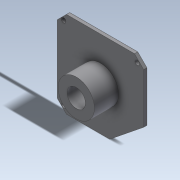
# Autodesk Inventor part: Arducam
Saved by Autodesk Inventor 2020 (Build 240168000, 168)
## iProperties
Created: 2020-11-17
Part Number: Arducam
Material: Generic
Document SubType Name: Modeling
Designer: valer
Density: 1 g/cm^3
Appearance: Default
Author: valer
Autodesk Inventor part; units mm, degrees
ref_plane "YZ Plane" through (0, 0, 0) normal (1, 0, 0) x (0, 1, 0)
ref_plane "XZ Plane" through (0, 0, 0) normal (0, 1, 0) x (-1, 0, 0)
ref_plane "XY Plane" through (0, 0, 0) normal (0, 0, 1) x (1, 0, 0)
sketch "Base" plane through (0, 0, 0) normal (0, 0, 1) x (1, 0, 0)
  line L0 (-20, 20) -> (20, 20)
  line L1 (20, 20) -> (20, -20)
  line L2 (20, -20) -> (-20, -20)
  line L3 (-20, -20) -> (-20, 20)
  line L4 (-15.74, 20) -> (-20, 15.74)
  line L5 (15.74, 20) -> (20, 15.74)
  line L6 (-17.02, 17.02) -> (17.02, 17.02) construction
  line L7 (17.02, 17.02) -> (17.02, -17.02) construction
  line L8 (17.02, -17.02) -> (-17.02, -17.02) construction
  line L9 (-17.02, -17.02) -> (-17.02, 17.02) construction
  line L10 (-17.02, 17.02) -> (17.02, -17.02) construction
  line L11 (17.02, 17.02) -> (-17.02, -17.02) construction
  circle A0 centre (0, 0) radius 8.4
  circle A1 centre (17.02, 17.02) radius 1.05
  circle A2 centre (-17.02, 17.02) radius 1.05
  circle A3 centre (-17.02, -17.02) radius 1.05
  circle A4 centre (17.02, -17.02) radius 1.05
  line L12 (-20, -15.74) -> (-15.74, -20)
  line L13 (20, -15.74) -> (15.74, -20)
  point P0 (0, 0)
  point P1 (0, 0)
  dimension "d0" = 40
  dimension "d1" = 40
  dimension "d2" = 135
  dimension "d3" = 135
  dimension "d4" = 31.48
  dimension "d5" = 34.04
  dimension "d6" = 2.98
  dimension "d7" = 2.98
  dimension "d8" = 2.98
  dimension "d9" = 2.98
  dimension "d10" = 16.8
  dimension "d11" = 2.1
  dimension "d12" = 135
  dimension "d13" = 135
  dimension "d14" = 31.48
  dimension "d15" = 34.04
  dimension "d16" = 31.48
  constraints: 28 end point, 8 point on line, 5 centre point, 5 coincident, 5 perpendicular, 4 parallel, 3 equal radius, 2 horizontal, 2 midpoint
  measures "d0" distance of L0.start L0.end
  measures "d1" distance of L2.end L0.start
  measures "d2" angle of L0 L4
  measures "d3" angle of L0 L5
  measures "d4" distance of L5.start L4.start
  measures "d5" distance of L6.start L6.end
  measures "d6" distance between parallel lines of L3 L9
  measures "d7" distance between parallel lines of L1 L7
  measures "d8" distance between parallel lines of L0 L6
  measures "d9" distance between parallel lines of L2 L8
  measures "d10" diameter of A0
  measures "d11" diameter of A1
  measures "d12" angle of L2 L12
  measures "d13" angle of L2 L13
  measures "d14" distance of L12.start L4.end
  measures "d15" distance of L8.end L6.start
  measures "d16" distance of L13.start L5.end
extrude "BaseFeature" add sketch "Base" along normal blind 1.5 contours L0 L5 L1 L13 L2 L12 L3 L4 | A0
extrude "CameraFeature" add sketch "Base" along normal blind 12.7 contours A0
sketch "Sketch2" plane through (0, 0, 12.7) normal (0, 0, 1) x (1, 0, 0)
  circle A0 centre (0, 0) radius 8.4 projected
  circle A1 centre (0, 0) radius 4.2489
  point P0 (0, 0)
  dimension "d21" = 4.151
  constraints: 1 centre point
  measures "d21" radial gap between concentric circles of A0 A1
extrude "Extrusion3" cut sketch "Sketch2" against normal blind 7.62 contours A1
sketch "Sketch3" plane through (0, 0, 1.5) normal (0, 0, 1) x (1, 0, 0)
  line L0 (20, -15.74) -> (20, 15.74) projected
  line L1 (20, -7.3568) -> (4.3044, -20)
  line L2 (-15.74, -20) -> (15.74, -20) projected
  line L3 (15.74, -20) -> (20, -15.74) projected
  line L4 (20, -15.74) -> (15.74, -20)
  point P0 (0, 0)
  dimension "d24" = 11.4356
  dimension "d25" = 8.3832
  constraints: 4 end point, 2 point on line, 1 collinear
  measures "d24" distance of L2.end L1.end
  measures "d25" distance of L1.start L0.start
extrude "Extrusion4" cut sketch "Sketch3" against normal through all
equation "\"d1\" = d0"
equation "\"d3\" = d2"
equation "\"d7\" = d6"
equation "\"d9\" = d8"
equation "\"d12\" = d2"
equation "\"d13\" = d2"
equation "\"d14\" = d4"
body "Solid1"
